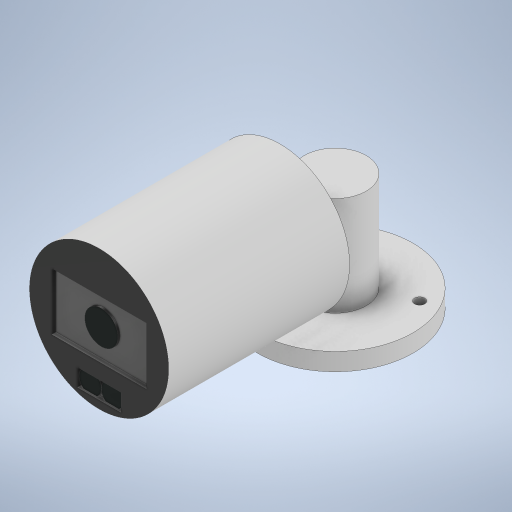
# Autodesk Inventor part: camera real
Saved by Autodesk Inventor 2024.1 (Build 281209000, 209)
## iProperties
Created: 2026-03-24
Part Number: camera real
Material: Generic
Document SubType Name: Modeling
Designer: User
Density: 1 g/cm^3
Appearance: Default
Author: User
Autodesk Inventor part; units mm, degrees
ref_plane "YZ Plane" through (0, 0, 0) normal (1, 0, 0) x (0, 1, 0)
ref_plane "XZ Plane" through (0, 0, 0) normal (0, 1, 0) x (-1, 0, 0)
ref_plane "XY Plane" through (0, 0, 0) normal (0, 0, 1) x (1, 0, 0)
sketch "Sketch1" plane through (0, 0, 0) normal (0, 1, 0) x (-1, 0, 0)
  circle A0 centre (0, 0) radius 35.2
  dimension "d0" = 70.4
  constraints: 1 centre point, 1 coincident
  measures "d0" diameter of A0
extrude "Extrusion1" add sketch "Sketch1" along normal blind 8
sketch "Sketch2" plane through (0, 8, 0) normal (0, 1, 0) x (1, 0, 0)
  circle A0 centre (0, 0) radius 14
  dimension "d3" = 28
  constraints: 1 centre point, 1 coincident
  measures "d3" diameter of A0
extrude "Extrusion2" add sketch "Sketch2" along normal blind 45
sketch "Sketch3" plane through (0, 0, 0) normal (0, 0, 1) x (1, 0, 0)
  circle A0 centre (0, 45.5) radius 7.5
  point P0 (0, 0)
  constraints: 1 centre point
extrude "Extrusion3" add sketch "Sketch3" along normal blind 25
sketch "Sketch4" plane through (0, 45.5, 25) normal (0, 0, 1) x (1, 0, 0)
  circle A0 centre (0, 0) radius 31.5
  point P0 (0, -45.5)
  dimension "d8" = 63
  constraints: 1 centre point
  measures "d8" diameter of A0
extrude "Extrusion4" add sketch "Sketch4" along normal blind 82
sketch "Sketch5" plane through (0, 45.5, 107) normal (0, 0, 1) x (1, 0, 0)
  line L0 (-21.5, 13) -> (21.5, 13)
  line L1 (21.5, 13) -> (21.5, -13)
  line L2 (21.5, -13) -> (-21.5, -13)
  line L3 (-21.5, -13) -> (-21.5, 13)
  line L4 (-21.5, 13) -> (21.5, -13) construction
  line L5 (21.5, 13) -> (-21.5, -13) construction
  line L6 (-10, -20) -> (10, -20)
  line L7 (10, -20) -> (10, -28)
  line L8 (10, -28) -> (-10, -28)
  line L9 (-10, -28) -> (-10, -20)
  line L10 (-10, -20) -> (10, -28) construction
  line L11 (10, -20) -> (-10, -28) construction
  point P0 (0, -45.5)
  point P1 (0, 0)
  point P2 (0, -24)
  dimension "d11" = 43
  dimension "d12" = 26
  dimension "d13" = 20
  dimension "d14" = 8
  constraints: 24 end point, 4 midpoint, 4 parallel, 2 horizontal, 2 perpendicular
  measures "d11" distance of L1.end L2.end
  measures "d12" distance of L0.end L1.end
  measures "d13" distance of L7.end L8.end
  measures "d14" distance of L6.end L7.end
extrude "Extrusion5" cut sketch "Sketch5" against normal blind 2
sketch "Sketch6" plane through (0, 45.5, 105) normal (0, 0, 1) x (1, 0, 0)
  circle A0 centre (0, 0) radius 7.5
  circle A1 centre (-5, -24) radius 5
  circle A2 centre (5, -24) radius 5
  point P0 (0, -45.5)
  point P1 (0, -24)
  dimension "d17" = 15
  dimension "d18" = 10
  dimension "d19" = 10
  constraints: 3 centre point
  measures "d17" diameter of A0
  measures "d18" diameter of A1
  measures "d19" diameter of A2
extrude "Extrusion6" add sketch "Sketch6" along normal blind 1
sketch "Sketch8" plane through (0, 0, 0) normal (0, -1, 0) x (1, 0, 0)
  circle A0 centre (0, 0) radius 28 construction
  line L0 (0, 0) -> (50, 0) construction
  line L1 (0, 0) -> (-43.3013, -25) construction
  line L2 (0, 0) -> (50, 0) construction
  line L3 (0, 0) -> (0, 50)
  line L4 (0, 0) -> (50, 0) construction
  circle A1 centre (0, 28) radius 2.3
  circle A2 centre (-24.2487, -14) radius 2.3
  line L5 (0, 0) -> (43.3013, -25) construction
  line L6 (0, 0) -> (50, 0) construction
  circle A3 centre (24.2487, -14) radius 2.3
  dimension "d22" = 56
  dimension "d26" = 50
  dimension "d27" = 210
  dimension "d28" = 50
  dimension "d29" = 90
  dimension "d30" = 4.6
  dimension "d31" = 4.6
  dimension "d34" = 50
  dimension "d35" = 30
  dimension "d36" = 4.6
  constraints: 14 end point, 4 centre point, 4 horizontal, 3 equal length, 3 point on circle, 3 point on line, 1 coincident
  measures "d22" diameter of A0
  measures "d26" distance of L0.start L1.end
  measures "d28" distance of L0.start L3.end
  measures "d29" angle of L4 L3
  measures "d30" diameter of A1
  measures "d31" diameter of A2
  measures "d34" distance of L0.start L5.end
  measures "d35" angle of L5 L6
  measures "d36" diameter of A3
extrude "Extrusion7" cut sketch "Sketch8" against normal blind 8
body "Solid1"
